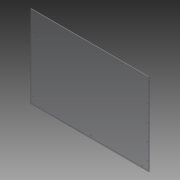
# Autodesk Inventor part: Hopper Top
Saved by Autodesk Inventor 2014 SP1 (Build 180222100, 222)
## iProperties
Created: 2013-12-16
Part Number: Hopper Top
Material: Polycarbonate, Clear
Document SubType Name: Modeling
Designer: Moses
Mass: 596.873 g
Surface Area: 3189.38 cm^2
Volume: 497.394 cm^3
Density: 1.2 g/cm^3
Appearance: Polycarbonate - Clear
Author: Moses
Autodesk Inventor part; units mm, degrees
ref_plane "YZ Plane" through (0, 0, 0) normal (1, 0, 0) x (0, 1, 0)
ref_plane "XZ Plane" through (0, 0, 0) normal (0, 1, 0) x (-1, 0, 0)
ref_plane "XY Plane" through (0, 0, 0) normal (0, 0, 1) x (1, 0, 0)
sketch "Sketch1" plane through (0, 0, 0) normal (0, 0, 1) x (1, 0, 0)
  line L0 (0, 0) -> (474.8218, 0)
  line L1 (474.8218, 0) -> (474.8218, 330.2)
  line L2 (474.8218, 330.2) -> (0, 330.2)
  line L3 (0, 330.2) -> (0, 0)
  circle A0 centre (467.2811, 231.775) radius 1.5875 projected
  circle A1 centre (467.2811, 98.425) radius 1.5875 projected
  circle A2 centre (467.2811, 31.75) radius 1.5875 projected
  circle A3 centre (467.2811, 165.1) radius 1.5875 projected
  circle A4 centre (467.2811, 298.45) radius 1.5875 projected
  line L4 (475.6155, 19.05) -> (459.7405, 19.05) construction
  line L5 (475.6155, 19.05) -> (475.6155, 311.15) construction
  line L6 (459.7405, 311.15) -> (475.6155, 311.15) construction
  line L7 (459.7405, 19.05) -> (459.7405, 311.15) construction
  circle A5 centre (7.5406, 97.6313) radius 1.5875 projected
  circle A6 centre (7.5406, 240.5063) radius 1.5875 projected
  circle A7 centre (7.5406, 311.9438) radius 1.5875 projected
  circle A8 centre (7.5406, 169.0688) radius 1.5875 projected
  circle A9 centre (7.5406, 26.1938) radius 1.5875 projected
  line L8 (-0.7937, 321.4688) -> (15.0813, 321.4688) construction
  line L9 (-0.7937, 321.4688) -> (-0.7937, 16.6688) construction
  line L10 (15.0813, 16.6688) -> (-0.7937, 16.6688) construction
  line L11 (15.0813, 321.4688) -> (15.0813, 16.6688) construction
  circle A10 centre (241.3, 7.5406) radius 1.5875 projected
  circle A11 centre (34.925, 7.5406) radius 1.5875 projected
  circle A12 centre (447.675, 7.5406) radius 1.5875 projected
  line L12 (25.4, -0.7938) -> (25.4, 15.0812) construction
  line L13 (25.4, -0.7938) -> (457.2, -0.7937) construction
  line L14 (457.2, 15.0813) -> (457.2, -0.7937) construction
  line L15 (25.4, 15.0812) -> (457.2, 15.0813) construction
  circle A13 centre (424.0218, 317.5) radius 1.5875
  circle A14 centre (322.4218, 317.5) radius 1.5875
  circle A15 centre (220.8218, 317.5) radius 1.5875
  dimension "d0" = 474.8218
  dimension "d1" = 330.2
  dimension "d4" = 3.175
  dimension "d7" = 101.6
  dimension "d12" = 12.7
  dimension "d13" = 50.8
  constraints: 8 end point, 3 centre point, 2 horizontal, 2 perpendicular, 1 coincident, 1 vertical, 4 other
  measures "d0" distance of L1.end L2.end
  measures "d1" distance of L2.end L0.start
  measures "d4" diameter of A13
  measures "d7" distance of A13.centre A14.centre
  measures "d12" distance from line of L2 A13.centre
  measures "d13" distance from line of L1 A13.centre
extrude "Extrusion1" add sketch "Sketch1" along normal blind 3.175
body "Solid1"
